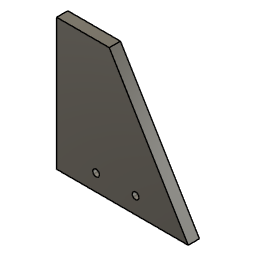
Tube Supporter v7 (Autodesk Fusion 360 design; units mm, degrees)
Autodesk Fusion 360 part; units mm, degrees
note: some values were not read from the file. Set by a fixed rule: which sketch regions a step uses.
sketch "Sketch1" plane through (0, 0, 0) normal (0, 0, 1) x (1, 0, 0)
  line L0 (0, 0) -> (0, 100)
  line L1 (0, 100) -> (40, 100)
  line L2 (40, 100) -> (100, 0)
  line L3 (100, 0) -> (0, 0)
  circle A0 centre (30, 12.5) radius 2.55
  circle A1 centre (60, 12.5) radius 2.55
  dimension "d3" = 40
  dimension "d4" = 100
  dimension "d5" = 100
  dimension "d14" = 12.5
  dimension "d15" = 12.5
  dimension "d16" = 5.1
  dimension "d17" = 5.1
  dimension "d18" = 30
  dimension "d19" = 30
  constraint coincident L0.start L3.end
  constraint vertical L0
  constraint perpendicular L0 L1
  constraint perpendicular L0 L3
  measures "d3" distance of L0.end L1.end
  measures "d4" distance of L0.start L0.end
  measures "d5" distance of L0.start L2.end
  measures "d14" distance of L3 A0.centre
  measures "d15" distance of L3 A1.centre
  measures "d16" diameter of A0
  measures "d17" diameter of A1
  measures "d18" distance of A0.centre A1.centre
  measures "d19" distance of L0 A0.centre
extrude "Extrude1" add sketch "Sketch1" along normal blind 8.5
equation "d15 = d14"
equation "d17 = d16"
